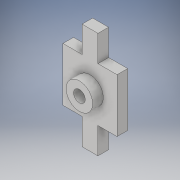
# Autodesk Inventor part: amt_plate
Saved by Autodesk Inventor 2019 (Build 230136000, 136)
## iProperties
Created: 2024-08-27
Part Number: amt_plate
Material: Generisch
Document SubType Name: Modeling
Designer: nic
Density: 1 g/cm^3
Appearance: Vorgabe
Author: nic
Autodesk Inventor part; units mm, degrees
ref_plane "YZ Plane" through (0, 0, 0) normal (1, 0, 0) x (0, 1, 0)
ref_plane "XZ Plane" through (0, 0, 0) normal (0, 1, 0) x (-1, 0, 0)
ref_plane "XY Plane" through (0, 0, 0) normal (0, 0, 1) x (1, 0, 0)
sketch "Skizze1" plane through (0, 0, 0) normal (0, 0, 1) x (1, 0, 0)
  line L0 (2.8537, 62.8557) -> (-11.3867, 62.8557) projected
  line L1 (-8.4337, 63.8875) -> (2.8537, 63.8875) projected
  line L2 (2.8537, 63.8875) -> (2.8537, 62.8557) projected
  line L3 (5.1, 52.7557) -> (-5.1, 52.7557)
  line L4 (-5.1, 52.7557) -> (-5.1, 72.9557)
  line L5 (-5.1, 72.9557) -> (5.1, 72.9557)
  line L6 (5.1, 72.9557) -> (5.1, 52.7557)
  line L7 (5.1, 52.7557) -> (-5.1, 72.9557) construction
  line L8 (-5.1, 52.7557) -> (5.1, 72.9557) construction
  line L9 (5.1, 62.8557) -> (-5.1, 62.8557)
  point P0 (0, 0)
  point P1 (0, 62.8557)
  constraints: 14 end point, 4 midpoint, 2 parallel, 1 horizontal, 1 perpendicular, 1 point on line
extrude "Extrusion1" add sketch "Skizze1" along normal blind 2 contours L0 L4 L1 L2 | L2 L1 L4 L5 L6 L9
sketch "Skizze2" plane through (0, 0, 2) normal (0, 0, 1) x (1, 0, 0)
  line L0 (-5.1, 72.9557) -> (-5.1, 62.8557) projected
  line L1 (-5.1, 62.8557) -> (5.1, 62.8557) projected
  line L2 (5.1, 62.8557) -> (5.1, 72.9557) projected
  line L3 (5.1, 72.9557) -> (-5.1, 72.9557) projected
  circle A0 centre (0, 67.9057) radius 2.5
  circle A1 centre (0, 67.9057) radius 1.1
  point P0 (0, 0)
  dimension "d4" = 5
  dimension "d5" = 2.2
  constraints: 2 centre point, 1 coincident
  measures "d4" diameter of A0
  measures "d5" diameter of A1
extrude "Extrusion2" add sketch "Skizze2" along normal blind 2 contours A0
sketch "Skizze3" plane through (0, 0, 2) normal (0, 0, 1) x (1, 0, 0)
  circle A0 centre (0, 67.9057) radius 1.1 projected
  point P0 (0, 0)
extrude "Extrusion3" cut sketch "Skizze3" against normal blind 2
sketch "Skizze4" plane through (0, 0, 0) normal (0, 0, -1) x (-1, 0, 0)
  circle A0 centre (0, 67.9057) radius 1.1 construction
  line L0 (1.5, 77.9057) -> (-1.5, 77.9057)
  line L1 (-1.5, 77.9057) -> (-1.5, 57.9057)
  line L2 (-1.5, 57.9057) -> (1.5, 57.9057)
  line L3 (1.5, 57.9057) -> (1.5, 77.9057)
  line L4 (1.5, 77.9057) -> (-1.5, 57.9057) construction
  line L5 (-1.5, 77.9057) -> (1.5, 57.9057) construction
  point P0 (0, 0)
  dimension "d10" = 3
  dimension "d11" = 20
  constraints: 12 end point, 2 midpoint, 2 parallel, 1 horizontal, 1 perpendicular
  measures "d10" distance of L2.end L1.end
  measures "d11" distance of L1.end L0.end
extrude "Extrusion4" add sketch "Skizze4" against normal blind 2
sketch "Skizze5" plane through (0, 0, 0) normal (0, 0, -1) x (-1, 0, 0)
  circle A0 centre (0, 67.9057) radius 1.1 projected
  point P0 (0, 0)
extrude "Extrusion5" cut sketch "Skizze5" against normal blind 10
